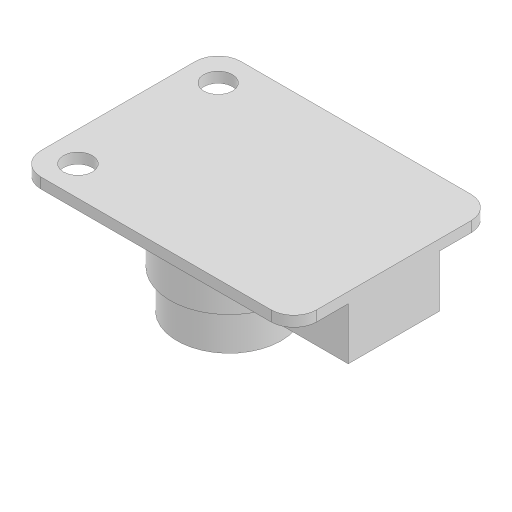
# Autodesk Inventor part: DF Robot DFR0029-R
Saved by Autodesk Inventor 2024.3 (Build 283343000, 343)
## iProperties
Created: 2025-08-19
Part Number: DF Robot DFR0029-R
Material: Generic
Document SubType Name: Modeling
Designer: PM
Density: 1 g/cm^3
Appearance: Default
Author: PM
Autodesk Inventor part; units mm, degrees
ref_plane "YZ Plane" through (0, 0, 0) normal (1, 0, 0) x (0, 1, 0)
ref_plane "XZ Plane" through (0, 0, 0) normal (0, 1, 0) x (-1, 0, 0)
ref_plane "XY Plane" through (0, 0, 0) normal (0, 0, 1) x (1, 0, 0)
sketch "Sketch1" plane through (0, 0, 0) normal (0, 1, 0) x (-1, 0, 0)
  line L0 (-15.1, 10.95) -> (15.1, 10.95)
  line L1 (15.1, 10.95) -> (15.1, -10.95)
  line L2 (15.1, -10.95) -> (-15.1, -10.95)
  line L3 (-15.1, -10.95) -> (-15.1, 10.95)
  line L4 (-15.1, 10.95) -> (15.1, -10.95) construction
  line L5 (15.1, 10.95) -> (-15.1, -10.95) construction
  line L6 (-3.5, 6.45) -> (9.4, 6.45)
  line L7 (9.4, 6.45) -> (9.4, -6.45)
  line L8 (9.4, -6.45) -> (-3.5, -6.45)
  line L9 (-3.5, -6.45) -> (-3.5, 6.45)
  line L10 (-3.5, 6.45) -> (9.4, -6.45) construction
  line L11 (9.4, 6.45) -> (-3.5, -6.45) construction
  circle A0 centre (2.95, 0) radius 6.45
  point P0 (0, 0)
  dimension "d0" = 21.9
  dimension "d1" = 30.2
  dimension "d3" = 12.9
  dimension "d4" = 18.6
  constraints: 24 end point, 4 midpoint, 4 parallel, 2 horizontal, 2 perpendicular, 2 tangent, 1 centre point, 1 coincident, 1 horizontal alignment
  measures "d0" distance of L0.end L1.end
  measures "d1" distance of L1.end L2.end
  measures "d3" diameter of A0
  measures "d4" distance between parallel lines of L1 L9
extrude "Extrusion1" add sketch "Sketch1" along normal blind 1.15 contours L0 L1 L2 L3 | L6 A0 L9 | L6 L7 A0 | A0 | A0 L8 L9 | L7 L8 A0
extrude "Extrusion2" add sketch "Sketch1" against normal blind 8 contours A0
sketch "Sketch2" plane through (0, -8, 0) normal (0, -1, 0) x (1, 0, 0)
  line L0 (3.5, -6.45) -> (3.5, 6.45) projected
  line L1 (3.5, 6.45) -> (-9.4, 6.45) projected
  line L2 (-9.4, 6.45) -> (-9.4, -6.45) projected
  line L3 (-9.4, -6.45) -> (3.5, -6.45) projected
  line L4 (3.5, 6.45) -> (-9.4, -6.45)
  line L5 (3.5, -6.45) -> (-9.4, 6.45)
  circle A0 centre (-2.95, 0) radius 5.7
  point P0 (0, 0)
  dimension "d9" = 11.4
  constraints: 4 end point, 1 centre point, 1 coincident, 1 midpoint, 1 perpendicular
  measures "d9" diameter of A0
extrude "Extrusion3" add sketch "Sketch2" along normal blind 4.2 contours A0 L4 L5 | L5 L4 A0 | L4 L5 A0 | A0 L5 L4
sketch "Sketch3" plane through (0, 0, 0) normal (0, -1, 0) x (1, 0, 0)
  line L0 (15.1, -10.95) -> (-15.1, -10.95) projected
  line L1 (15.1, 10.95) -> (15.1, -10.95) projected
  line L2 (-15.1, 10.95) -> (15.1, 10.95) projected
  line L3 (-15.1, -10.95) -> (-15.1, 10.95) projected
  line L4 (15.1, -5) -> (7.1, -5)
  line L5 (7.1, -5) -> (7.1, 5)
  line L6 (7.1, 5) -> (15.1, 5)
  line L7 (15.1, 5) -> (15.1, -5)
  line L8 (15.1, -5) -> (7.1, 5) construction
  line L9 (7.1, -5) -> (15.1, 5) construction
  line L10 (15.1, 10.95) -> (15.1, -10.95) projected
  point P0 (0, 0)
  point P1 (11.1, 0)
  point P2 (15.1, 0)
  dimension "d12" = 10
  dimension "d13" = 8
  constraints: 12 end point, 3 midpoint, 2 parallel, 1 horizontal, 1 horizontal alignment, 1 perpendicular, 1 point on line
  measures "d12" distance of L4.end L5.end
  measures "d13" distance of L5.end L6.end
extrude "Extrusion4" add sketch "Sketch3" along normal blind 5.7 contours L4 L5 L6 L1
sketch "Sketch4" plane through (0, 0, 0) normal (0, -1, 0) x (1, 0, 0)
  line L0 (7.1, 5) -> (15.1, 5) projected
  line L1 (15.1, 10.95) -> (15.1, 5) projected
  line L2 (-15.1, 10.95) -> (15.1, 10.95) projected
  line L3 (-15.1, -10.95) -> (-15.1, 10.95) projected
  line L4 (15.1, -10.95) -> (-15.1, -10.95) projected
  line L5 (15.1, -5) -> (15.1, -10.95) projected
  line L6 (15.1, -5) -> (7.1, -5) projected
  line L7 (7.1, -5) -> (7.1, 5) projected
  circle A0 centre (-11.825, -7.675) radius 1.575
  circle A1 centre (-11.825, 7.675) radius 1.575
  line L8 (-10.25, -9.6033) -> (-10.25, -6.1)
  line L9 (-10.25, -6.1) -> (-13.9455, -6.1)
  point P0 (0, 0)
  dimension "d16" = 3.15
  dimension "d17" = 3.15
  dimension "d18" = 4.85
  dimension "d19" = 3.275
  dimension "d20" = 3.275
  dimension "d21" = 4.85
  constraints: 4 end point, 2 centre point, 2 coincident, 2 tangent, 1 perpendicular, 1 vertical, 1 vertical alignment
  measures "d16" diameter of A0
  measures "d17" diameter of A1
  measures "d18" distance between parallel lines of L4 L9
  measures "d19" distance from line of L4 point (-11.825, -7.675)
  measures "d20" distance from line of L2 A1.centre
  measures "d21" distance between parallel lines of L3 L8
extrude "Extrusion5" cut sketch "Sketch4" against normal through all contours A0 | A1
fillet "Fillet1" radius 2.5 4 edges at (-15.1, 0.575, -10.95) (-15.1, 0.575, 10.95) (15.1, 0.575, -10.95) (15.1, 0.575, 10.95)
sketch "Sketch5" plane through (0, 0, 0) normal (0, -1, 0) x (1, 0, 0)
  circle A0 centre (-11.825, 7.675) radius 1.575 projected
  circle A1 centre (-11.825, -7.675) radius 1.575 projected
  arc A2 (15.1, 8.45) -> (12.6, 10.95) centre (12.6, 8.45) ccw projected
  line L0 (-12.6, 10.95) -> (12.6, 10.95) projected
  arc A3 (-12.6, 10.95) -> (-15.1, 8.45) centre (-12.6, 8.45) ccw projected
  line L1 (-15.1, -8.45) -> (-15.1, 8.45) projected
  arc A4 (-15.1, -8.45) -> (-12.6, -10.95) centre (-12.6, -8.45) ccw projected
  line L2 (12.6, -10.95) -> (-12.6, -10.95) projected
  arc A5 (12.6, -10.95) -> (15.1, -8.45) centre (12.6, -8.45) ccw projected
  line L3 (15.1, -5) -> (15.1, -8.45) projected
  line L4 (15.1, -5) -> (7.1, -5) projected
  line L5 (7.1, -5) -> (7.1, 5) projected
  line L6 (7.1, 5) -> (15.1, 5) projected
  line L7 (15.1, 8.45) -> (15.1, 5) projected
  line L8 (-15.1, -8.45) -> (-15.1, -10.95)
  line L9 (-15.1, -10.95) -> (-12.6, -10.95)
  line L10 (-14.9891, 11.1013) -> (15.1, 10.95) construction
  line L11 (15.1, 10.95) -> (14.9891, -11.1013) construction
  line L12 (14.9891, -11.1013) -> (-15.1, -10.95) construction
  line L13 (-15.1, -10.95) -> (-14.9891, 11.1013) construction
  line L14 (12.6, 10.95) -> (15.1, 10.95)
  line L15 (15.1, 10.95) -> (15.1, 8.45)
  point P0 (0, 0)
  constraints: 8 end point, 2 coincident, 2 perpendicular, 2 tangent, 1 horizontal, 1 vertical, 2 other
decal "Decal1"
decal "Decal2"
decal "Decal3"
decal "Decal4"
equation "\"d20\" = d19"
equation "\"d21\" = d18"
body "Solid1"
